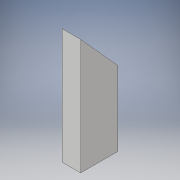
# Autodesk Inventor part: SmallAnglesSupport.ver1-1111-2020
Saved by Autodesk Inventor 2018 (Build 220112000, 112)
## iProperties
Created: 2020-01-19
Part Number: SmallAnglesSupport.ver1-1111-2020
Material: Generic
Document SubType Name: Modeling
Designer: JMHal
Density: 1 g/cm^3
Appearance: Default
Author: JMHal
Autodesk Inventor part; units mm, degrees
ref_plane "YZ Plane" through (0, 0, 0) normal (1, 0, 0) x (0, 1, 0)
ref_plane "XZ Plane" through (0, 0, 0) normal (0, 1, 0) x (-1, 0, 0)
ref_plane "XY Plane" through (0, 0, 0) normal (0, 0, 1) x (1, 0, 0)
sketch "Sketch1" plane through (0, 0, 0) normal (0, 1, 0) x (-1, 0, 0)
  line L0 (0, 0) -> (25.4, 0)
  line L1 (25.4, 0) -> (25.4, -50.8)
  line L2 (25.4, -50.8) -> (0, -50.8)
  line L3 (0, -50.8) -> (0, 0)
  line L4 (22.225, -47.625) -> (22.225, -3.175)
  line L5 (22.225, -3.175) -> (3.175, -3.175)
  line L6 (3.175, -3.175) -> (3.175, -47.625)
  line L7 (3.175, -47.625) -> (22.225, -47.625)
  dimension "d0" = 25.4
  dimension "d1" = 50.8
  dimension "d2" = 3.175
  constraints: 16 end point, 4 parallel, 2 perpendicular, 1 horizontal, 3 other
  measures "d0" distance of L1.end L2.end
  measures "d1" distance of L0.end L1.end
  measures "d2" distance between parallel lines of L1 L4
extrude "Extrusion1" add sketch "Sketch1" along normal blind 75.4888
sketch "Sketch2" plane through (0, 0, 0) normal (1, 0, 0) x (0, 0, -1)
  line L0 (50.8, 0) -> (0, 0) projected
  line L1 (50.8, 0) -> (50.8, 75.4888) projected
  line L2 (0, 75.4888) -> (50.8, 75.4888) projected
  line L3 (0, 0) -> (0, 75.4888) projected
  line L4 (50.8, 75.4888) -> (0, 131.9079)
  line L5 (0, 131.9079) -> (0, 75.4888)
  dimension "d5" = 48
  constraints: 4 end point, 1 collinear
  measures "d5" angle of L4 L2
extrude "Extrusion2" add sketch "Sketch2" against normal blind 25.4 contours L2 L5 L4
sketch "Sketch3" plane through (0, 0, 0) normal (0, -1, 0) x (1, 0, 0)
  line L0 (-22.225, -47.625) -> (-3.175, -47.625) projected
  line L1 (-3.175, -47.625) -> (-3.175, -3.175) projected
  line L2 (-3.175, -3.175) -> (-22.225, -3.175) projected
  line L3 (-22.225, -3.175) -> (-22.225, -47.625) projected
  point P0 (0, 0)
extrude "Extrusion3" cut sketch "Sketch3" against normal through all
sketch "Sketch4" plane through (0, 0, 0) normal (0, -1, 0) x (1, 0, 0)
  line L0 (-3.175, -47.625) -> (-22.225, -47.625) projected
  line L1 (-22.225, -47.625) -> (-22.225, -3.175) projected
  line L2 (-22.225, -3.175) -> (-3.175, -3.175) projected
  line L3 (-3.175, -3.175) -> (-3.175, -47.625) projected
  line L4 (0, 0) -> (-25.4, 0) projected
  line L5 (-25.4, 0) -> (-25.4, -50.8) projected
  line L6 (-25.4, -50.8) -> (0, -50.8) projected
  line L7 (0, -50.8) -> (0, 0) projected
extrude "Extrusion4" add sketch "Sketch4" along normal blind 25.4
body "Solid1"
